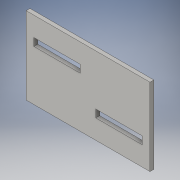
# Autodesk Inventor part: vexPlate
Saved by Autodesk Inventor 2016 SP1 (Build 200210100, 210)
## iProperties
Created: 2015-11-22
Part Number: vexPlate
Material: Generic
Document SubType Name: Modeling
Designer: steele
Density: 1 g/cm^3
Appearance: Default
Author: steele
Autodesk Inventor part; units mm, degrees
ref_plane "YZ Plane" through (0, 0, 0) normal (1, 0, 0) x (0, 1, 0)
ref_plane "XZ Plane" through (0, 0, 0) normal (0, 1, 0) x (-1, 0, 0)
ref_plane "XY Plane" through (0, 0, 0) normal (0, 0, 1) x (1, 0, 0)
sketch "Sketch1" plane through (0, 0, 0) normal (0, 0, 1) x (1, 0, 0)
  line L0 (-101.6, -63.5) -> (101.6, -63.5)
  line L1 (101.6, -63.5) -> (101.6, 63.5)
  line L2 (101.6, 63.5) -> (-101.6, 63.5)
  line L3 (-101.6, 63.5) -> (-101.6, -63.5)
  line L4 (-12.7, 63.5) -> (-12.7, -63.5) construction
  line L5 (12.7, 63.5) -> (12.7, -63.5) construction
  line L6 (-101.6, 25.4) -> (101.6, 25.4) construction
  line L7 (-101.6, -25.4) -> (101.6, -25.4) construction
  line L8 (-50.8, 63.5) -> (-50.8, -63.5) construction
  line L9 (50.8, 63.5) -> (50.8, -63.5) construction
  line L10 (-88.9, 19.05) -> (-12.7, 19.05)
  line L11 (-12.7, 19.05) -> (-12.7, 31.75)
  line L12 (-12.7, 31.75) -> (-88.9, 31.75)
  line L13 (-88.9, 31.75) -> (-88.9, 19.05)
  line L14 (-88.9, 19.05) -> (-12.7, 31.75) construction
  line L15 (-12.7, 19.05) -> (-88.9, 31.75) construction
  line L16 (12.7, -31.75) -> (88.9, -31.75)
  line L17 (88.9, -31.75) -> (88.9, -19.05)
  line L18 (88.9, -19.05) -> (12.7, -19.05)
  line L19 (12.7, -19.05) -> (12.7, -31.75)
  line L20 (12.7, -31.75) -> (88.9, -19.05) construction
  line L21 (88.9, -31.75) -> (12.7, -19.05) construction
  point P0 (0, 0)
  point P1 (-50.8, 25.4)
  point P2 (50.8, -25.4)
  dimension "d2" = 12.7
  dimension "d3" = 12.7
  dimension "d4" = 25.4
  dimension "d5" = 25.4
  dimension "d6" = 50.8
  dimension "d7" = 50.8
  dimension "d9" = 12.7
  dimension "d10" = 76.2
  dimension "d11" = 101.6
  dimension "d12" = 63.5
  dimension "d15" = 101.6
  dimension "d16" = 63.5
  constraints: 44 end point, 16 point on line, 10 parallel, 9 perpendicular, 4 midpoint, 1 horizontal
  measures "d2" distance from line of L4 point (0, 0)
  measures "d3" distance from line of point (0, 0) L5
  measures "d4" distance from line of point (0, 0) L6
  measures "d5" distance from line of point (0, 0) L7
  measures "d6" distance from line of L8 point (0, 0)
  measures "d7" distance from line of point (0, 0) L9
  measures "d9" distance of L12.end L10.start
  measures "d10" distance of L11.end L12.end
  measures "d11" distance from line of point (0, 0) L3
  measures "d12" distance from line of point (0, 0) L2
  measures "d15" distance from line of point (0, 0) L1
  measures "d16" distance from line of point (0, 0) L0
extrude "Extrusion1" add sketch "Sketch1" against normal blind 6.35
equation "\"d2\" = offsetForBracketHoles"
equation "\"d3\" = offsetForBracketHoles"
equation "\"d4\" = verticalCenterLineOfSlot"
equation "\"d5\" = verticalCenterLineOfSlot"
equation "\"d6\" = horizontalCenterLineOfSlot"
equation "\"d7\" = horizontalCenterLineOfSlot"
equation "\"d9\" = slotWidth"
equation "\"d10\" = slotLength"
equation "\"d11\" = 0.5 * plateWidth"
equation "\"d12\" = 0.5 * plateHeight"
equation "\"d15\" = 0.5 * plateWidth"
equation "\"d16\" = 0.5 * plateHeight"
equation "\"d13\" = plateThickness"
equation "\"plateWidth\" = 2 * offsetForBracketHoles + 2 * slotLength + 2 * edgeForSlot"
equation "\"plateHeight\" = 127"
equation "\"offsetForBracketHoles\" = 12.7"
equation "\"slotWidth\" = 12.7"
equation "\"slotLength\" = 76.2"
equation "\"verticalCenterLineOfSlot\" = 25.4"
equation "\"cylinderDiameter\" = 12.7"
equation "\"centerLineOfBracket\" = 17.526"
equation "\"horizontalCenterLineOfSlot\" = 0.5 * slotLength + offsetForBracketHoles"
equation "\"plateThickness\" = 6.35"
equation "\"edgeForSlot\" = 12.7"
body "Solid1"
